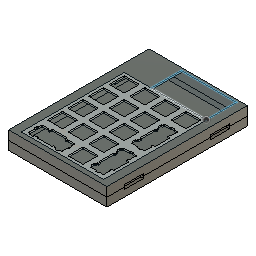
Keypad_case_top.glb (Autodesk Fusion 360 design; units mm, degrees)
part number: 2026-03-14-15-34-49-794
Autodesk Fusion 360 part; units mm, degrees
sketch "plate-2026-03-14T12_30_48.616Z" plane through (0, 0, 0) normal (0, 0, 1) x (1, 0, 0)
  line L0 (3.025, -26.3375) -> (16.025, -26.3375)
  line L1 (3.025, -40.3375) -> (16.025, -40.3375)
  line L2 (2.525, -26.8375) -> (2.525, -39.8375)
  line L3 (16.525, -26.8375) -> (16.525, -39.8375)
  arc A0 (3.025, -26.3375) -> (2.525, -26.8375) centre (3.025, -26.8375) ccw
  arc A1 (16.525, -26.8375) -> (16.025, -26.3375) centre (16.025, -26.8375) ccw
  arc A2 (2.525, -39.8375) -> (3.025, -40.3375) centre (3.025, -39.8375) ccw
  arc A3 (16.025, -40.3375) -> (16.525, -39.8375) centre (16.025, -39.8375) ccw
  line L4 (22.075, -26.3375) -> (35.075, -26.3375)
  line L5 (22.075, -40.3375) -> (35.075, -40.3375)
  line L6 (21.575, -26.8375) -> (21.575, -39.8375)
  line L7 (35.575, -26.8375) -> (35.575, -39.8375)
  arc A4 (22.075, -26.3375) -> (21.575, -26.8375) centre (22.075, -26.8375) ccw
  arc A5 (35.575, -26.8375) -> (35.075, -26.3375) centre (35.075, -26.8375) ccw
  arc A6 (21.575, -39.8375) -> (22.075, -40.3375) centre (22.075, -39.8375) ccw
  arc A7 (35.075, -40.3375) -> (35.575, -39.8375) centre (35.075, -39.8375) ccw
  line L8 (41.125, -26.3375) -> (54.125, -26.3375)
  line L9 (41.125, -40.3375) -> (54.125, -40.3375)
  line L10 (40.625, -26.8375) -> (40.625, -39.8375)
  line L11 (54.625, -26.8375) -> (54.625, -39.8375)
  arc A8 (41.125, -26.3375) -> (40.625, -26.8375) centre (41.125, -26.8375) ccw
  arc A9 (54.625, -26.8375) -> (54.125, -26.3375) centre (54.125, -26.8375) ccw
  arc A10 (40.625, -39.8375) -> (41.125, -40.3375) centre (41.125, -39.8375) ccw
  arc A11 (54.125, -40.3375) -> (54.625, -39.8375) centre (54.125, -39.8375) ccw
  line L12 (60.175, -26.3375) -> (73.175, -26.3375)
  line L13 (60.175, -40.3375) -> (73.175, -40.3375)
  line L14 (59.675, -26.8375) -> (59.675, -39.8375)
  line L15 (73.675, -26.8375) -> (73.675, -39.8375)
  arc A12 (60.175, -26.3375) -> (59.675, -26.8375) centre (60.175, -26.8375) ccw
  arc A13 (73.675, -26.8375) -> (73.175, -26.3375) centre (73.175, -26.8375) ccw
  arc A14 (59.675, -39.8375) -> (60.175, -40.3375) centre (60.175, -39.8375) ccw
  arc A15 (73.175, -40.3375) -> (73.675, -39.8375) centre (73.175, -39.8375) ccw
  line L16 (3.025, -45.3875) -> (16.025, -45.3875)
  line L17 (3.025, -59.3875) -> (16.025, -59.3875)
  line L18 (2.525, -45.8875) -> (2.525, -58.8875)
  line L19 (16.525, -45.8875) -> (16.525, -58.8875)
  arc A16 (3.025, -45.3875) -> (2.525, -45.8875) centre (3.025, -45.8875) ccw
  arc A17 (16.525, -45.8875) -> (16.025, -45.3875) centre (16.025, -45.8875) ccw
  arc A18 (2.525, -58.8875) -> (3.025, -59.3875) centre (3.025, -58.8875) ccw
  arc A19 (16.025, -59.3875) -> (16.525, -58.8875) centre (16.025, -58.8875) ccw
  line L20 (22.075, -45.3875) -> (35.075, -45.3875)
  line L21 (22.075, -59.3875) -> (35.075, -59.3875)
  line L22 (21.575, -45.8875) -> (21.575, -58.8875)
  line L23 (35.575, -45.8875) -> (35.575, -58.8875)
  arc A20 (22.075, -45.3875) -> (21.575, -45.8875) centre (22.075, -45.8875) ccw
  arc A21 (35.575, -45.8875) -> (35.075, -45.3875) centre (35.075, -45.8875) ccw
  arc A22 (21.575, -58.8875) -> (22.075, -59.3875) centre (22.075, -58.8875) ccw
  arc A23 (35.075, -59.3875) -> (35.575, -58.8875) centre (35.075, -58.8875) ccw
  line L24 (41.125, -45.3875) -> (54.125, -45.3875)
  line L25 (41.125, -59.3875) -> (54.125, -59.3875)
  line L26 (40.625, -45.8875) -> (40.625, -58.8875)
  line L27 (54.625, -45.8875) -> (54.625, -58.8875)
  arc A24 (41.125, -45.3875) -> (40.625, -45.8875) centre (41.125, -45.8875) ccw
  arc A25 (54.625, -45.8875) -> (54.125, -45.3875) centre (54.125, -45.8875) ccw
  arc A26 (40.625, -58.8875) -> (41.125, -59.3875) centre (41.125, -58.8875) ccw
  arc A27 (54.125, -59.3875) -> (54.625, -58.8875) centre (54.125, -58.8875) ccw
  line L28 (73.675, -55.4125) -> (73.675, -68.4125)
  line L29 (59.675, -55.4125) -> (59.675, -68.4125)
  line L30 (73.175, -54.9125) -> (60.175, -54.9125)
  line L31 (73.175, -68.9125) -> (60.175, -68.9125)
  arc A28 (73.675, -55.4125) -> (73.175, -54.9125) centre (73.175, -55.4125) ccw
  arc A29 (73.175, -68.9125) -> (73.675, -68.4125) centre (73.175, -68.4125) ccw
  arc A30 (60.175, -54.9125) -> (59.675, -55.4125) centre (60.175, -55.4125) ccw
  arc A31 (59.675, -68.4125) -> (60.175, -68.9125) centre (60.175, -68.4125) ccw
  line L32 (72.3646, -47.1471) -> (72.3646, -52.8019)
  line L33 (71.8646, -53.3019) -> (71.5518, -53.3019)
  line L34 (71.5518, -53.3019) -> (71.5518, -61.9125)
  line L35 (60.8584, -61.9125) -> (60.8584, -53.8019)
  line L36 (60.3584, -53.3019) -> (60.071, -53.3019)
  line L37 (60.071, -53.3019) -> (60.071, -51.9985)
  line L38 (59.571, -51.4985) -> (59.4026, -51.4985)
  line L39 (58.9026, -50.9985) -> (58.9026, -48.9505)
  line L40 (59.4026, -48.4505) -> (59.571, -48.4505)
  line L41 (60.071, -47.9505) -> (60.071, -47.1471)
  line L42 (60.571, -46.6471) -> (65.667, -46.6471)
  line L43 (66.167, -46.1471) -> (66.167, -45.7835)
  line L44 (66.167, -45.7835) -> (68.461, -45.7835)
  line L45 (68.961, -46.2835) -> (68.961, -46.6471)
  line L46 (68.961, -46.6471) -> (71.8646, -46.6471)
  arc A32 (71.8646, -53.3019) -> (72.3646, -52.8019) centre (71.8646, -52.8019) ccw
  arc A33 (60.8584, -53.8019) -> (60.3584, -53.3019) centre (60.3584, -53.8019) ccw
  arc A34 (60.071, -51.9985) -> (59.571, -51.4985) centre (59.571, -51.9985) ccw
  arc A35 (58.9026, -50.9985) -> (59.4026, -51.4985) centre (59.4026, -50.9985) ccw
  arc A36 (59.4026, -48.4505) -> (58.9026, -48.9505) centre (59.4026, -48.9505) ccw
  arc A37 (59.571, -48.4505) -> (60.071, -47.9505) centre (59.571, -47.9505) ccw
  arc A38 (60.571, -46.6471) -> (60.071, -47.1471) centre (60.571, -47.1471) ccw
  arc A39 (65.667, -46.6471) -> (66.167, -46.1471) centre (65.667, -46.1471) ccw
  arc A40 (68.961, -46.2835) -> (68.461, -45.7835) centre (68.461, -46.2835) ccw
  arc A41 (72.3646, -47.1471) -> (71.8646, -46.6471) centre (71.8646, -47.1471) ccw
  line L47 (72.3646, -76.6779) -> (72.3646, -71.0231)
  line L48 (71.8646, -70.5231) -> (71.5518, -70.5231)
  line L49 (71.5518, -70.5231) -> (71.5518, -61.9125)
  line L50 (60.8584, -61.9125) -> (60.8584, -70.0231)
  line L51 (60.3584, -70.5231) -> (60.071, -70.5231)
  line L52 (60.071, -70.5231) -> (60.071, -71.8265)
  line L53 (59.571, -72.3265) -> (59.4026, -72.3265)
  line L54 (58.9026, -72.8265) -> (58.9026, -74.8745)
  line L55 (59.4026, -75.3745) -> (59.571, -75.3745)
  line L56 (60.071, -75.8745) -> (60.071, -76.6779)
  line L57 (60.571, -77.1779) -> (65.667, -77.1779)
  line L58 (66.167, -77.6779) -> (66.167, -78.0415)
  line L59 (66.167, -78.0415) -> (68.461, -78.0415)
  line L60 (68.961, -77.5415) -> (68.961, -77.1779)
  line L61 (68.961, -77.1779) -> (71.8646, -77.1779)
  arc A42 (72.3646, -71.0231) -> (71.8646, -70.5231) centre (71.8646, -71.0231) ccw
  arc A43 (60.3584, -70.5231) -> (60.8584, -70.0231) centre (60.3584, -70.0231) ccw
  arc A44 (59.571, -72.3265) -> (60.071, -71.8265) centre (59.571, -71.8265) ccw
  arc A45 (59.4026, -72.3265) -> (58.9026, -72.8265) centre (59.4026, -72.8265) ccw
  arc A46 (58.9026, -74.8745) -> (59.4026, -75.3745) centre (59.4026, -74.8745) ccw
  arc A47 (60.071, -75.8745) -> (59.571, -75.3745) centre (59.571, -75.8745) ccw
  arc A48 (60.071, -76.6779) -> (60.571, -77.1779) centre (60.571, -76.6779) ccw
  arc A49 (66.167, -77.6779) -> (65.667, -77.1779) centre (65.667, -77.6779) ccw
  arc A50 (68.461, -78.0415) -> (68.961, -77.5415) centre (68.461, -77.5415) ccw
  arc A51 (71.8646, -77.1779) -> (72.3646, -76.6779) centre (71.8646, -76.6779) ccw
  line L62 (3.025, -64.4375) -> (16.025, -64.4375)
  line L63 (3.025, -78.4375) -> (16.025, -78.4375)
  line L64 (2.525, -64.9375) -> (2.525, -77.9375)
  line L65 (16.525, -64.9375) -> (16.525, -77.9375)
  arc A52 (3.025, -64.4375) -> (2.525, -64.9375) centre (3.025, -64.9375) ccw
  arc A53 (16.525, -64.9375) -> (16.025, -64.4375) centre (16.025, -64.9375) ccw
  arc A54 (2.525, -77.9375) -> (3.025, -78.4375) centre (3.025, -77.9375) ccw
  arc A55 (16.025, -78.4375) -> (16.525, -77.9375) centre (16.025, -77.9375) ccw
  line L66 (22.075, -64.4375) -> (35.075, -64.4375)
  line L67 (22.075, -78.4375) -> (35.075, -78.4375)
  line L68 (21.575, -64.9375) -> (21.575, -77.9375)
  line L69 (35.575, -64.9375) -> (35.575, -77.9375)
  arc A56 (22.075, -64.4375) -> (21.575, -64.9375) centre (22.075, -64.9375) ccw
  arc A57 (35.575, -64.9375) -> (35.075, -64.4375) centre (35.075, -64.9375) ccw
  arc A58 (21.575, -77.9375) -> (22.075, -78.4375) centre (22.075, -77.9375) ccw
  arc A59 (35.075, -78.4375) -> (35.575, -77.9375) centre (35.075, -77.9375) ccw
  line L70 (41.125, -64.4375) -> (54.125, -64.4375)
  line L71 (41.125, -78.4375) -> (54.125, -78.4375)
  line L72 (40.625, -64.9375) -> (40.625, -77.9375)
  line L73 (54.625, -64.9375) -> (54.625, -77.9375)
  arc A60 (41.125, -64.4375) -> (40.625, -64.9375) centre (41.125, -64.9375) ccw
  arc A61 (54.625, -64.9375) -> (54.125, -64.4375) centre (54.125, -64.9375) ccw
  arc A62 (40.625, -77.9375) -> (41.125, -78.4375) centre (41.125, -77.9375) ccw
  arc A63 (54.125, -78.4375) -> (54.625, -77.9375) centre (54.125, -77.9375) ccw
  line L74 (3.025, -83.4875) -> (16.025, -83.4875)
  line L75 (3.025, -97.4875) -> (16.025, -97.4875)
  line L76 (2.525, -83.9875) -> (2.525, -96.9875)
  line L77 (16.525, -83.9875) -> (16.525, -96.9875)
  arc A64 (3.025, -83.4875) -> (2.525, -83.9875) centre (3.025, -83.9875) ccw
  arc A65 (16.525, -83.9875) -> (16.025, -83.4875) centre (16.025, -83.9875) ccw
  arc A66 (2.525, -96.9875) -> (3.025, -97.4875) centre (3.025, -96.9875) ccw
  arc A67 (16.025, -97.4875) -> (16.525, -96.9875) centre (16.025, -96.9875) ccw
  line L78 (22.075, -83.4875) -> (35.075, -83.4875)
  line L79 (22.075, -97.4875) -> (35.075, -97.4875)
  line L80 (21.575, -83.9875) -> (21.575, -96.9875)
  line L81 (35.575, -83.9875) -> (35.575, -96.9875)
  arc A68 (22.075, -83.4875) -> (21.575, -83.9875) centre (22.075, -83.9875) ccw
  arc A69 (35.575, -83.9875) -> (35.075, -83.4875) centre (35.075, -83.9875) ccw
  arc A70 (21.575, -96.9875) -> (22.075, -97.4875) centre (22.075, -96.9875) ccw
  arc A71 (35.075, -97.4875) -> (35.575, -96.9875) centre (35.075, -96.9875) ccw
  line L82 (41.125, -83.4875) -> (54.125, -83.4875)
  line L83 (41.125, -97.4875) -> (54.125, -97.4875)
  line L84 (40.625, -83.9875) -> (40.625, -96.9875)
  line L85 (54.625, -83.9875) -> (54.625, -96.9875)
  arc A72 (41.125, -83.4875) -> (40.625, -83.9875) centre (41.125, -83.9875) ccw
  arc A73 (54.625, -83.9875) -> (54.125, -83.4875) centre (54.125, -83.9875) ccw
  arc A74 (40.625, -96.9875) -> (41.125, -97.4875) centre (41.125, -96.9875) ccw
  arc A75 (54.125, -97.4875) -> (54.625, -96.9875) centre (54.125, -96.9875) ccw
  line L86 (73.675, -93.5125) -> (73.675, -106.5125)
  line L87 (59.675, -93.5125) -> (59.675, -106.5125)
  line L88 (73.175, -93.0125) -> (60.175, -93.0125)
  line L89 (73.175, -107.0125) -> (60.175, -107.0125)
  arc A76 (73.675, -93.5125) -> (73.175, -93.0125) centre (73.175, -93.5125) ccw
  arc A77 (73.175, -107.0125) -> (73.675, -106.5125) centre (73.175, -106.5125) ccw
  arc A78 (60.175, -93.0125) -> (59.675, -93.5125) centre (60.175, -93.5125) ccw
  arc A79 (59.675, -106.5125) -> (60.175, -107.0125) centre (60.175, -106.5125) ccw
  line L90 (72.3646, -85.2471) -> (72.3646, -90.9019)
  line L91 (71.8646, -91.4019) -> (71.5518, -91.4019)
  line L92 (71.5518, -91.4019) -> (71.5518, -100.0125)
  line L93 (60.8584, -100.0125) -> (60.8584, -91.9019)
  line L94 (60.3584, -91.4019) -> (60.071, -91.4019)
  line L95 (60.071, -91.4019) -> (60.071, -90.0985)
  line L96 (59.571, -89.5985) -> (59.4026, -89.5985)
  line L97 (58.9026, -89.0985) -> (58.9026, -87.0505)
  line L98 (59.4026, -86.5505) -> (59.571, -86.5505)
  line L99 (60.071, -86.0505) -> (60.071, -85.2471)
  line L100 (60.571, -84.7471) -> (65.667, -84.7471)
  line L101 (66.167, -84.2471) -> (66.167, -83.8835)
  line L102 (66.167, -83.8835) -> (68.461, -83.8835)
  line L103 (68.961, -84.3835) -> (68.961, -84.7471)
  line L104 (68.961, -84.7471) -> (71.8646, -84.7471)
  arc A80 (71.8646, -91.4019) -> (72.3646, -90.9019) centre (71.8646, -90.9019) ccw
  arc A81 (60.8584, -91.9019) -> (60.3584, -91.4019) centre (60.3584, -91.9019) ccw
  arc A82 (60.071, -90.0985) -> (59.571, -89.5985) centre (59.571, -90.0985) ccw
  arc A83 (58.9026, -89.0985) -> (59.4026, -89.5985) centre (59.4026, -89.0985) ccw
  arc A84 (59.4026, -86.5505) -> (58.9026, -87.0505) centre (59.4026, -87.0505) ccw
  arc A85 (59.571, -86.5505) -> (60.071, -86.0505) centre (59.571, -86.0505) ccw
  arc A86 (60.571, -84.7471) -> (60.071, -85.2471) centre (60.571, -85.2471) ccw
  arc A87 (65.667, -84.7471) -> (66.167, -84.2471) centre (65.667, -84.2471) ccw
  arc A88 (68.961, -84.3835) -> (68.461, -83.8835) centre (68.461, -84.3835) ccw
  arc A89 (72.3646, -85.2471) -> (71.8646, -84.7471) centre (71.8646, -85.2471) ccw
  line L105 (72.3646, -114.7779) -> (72.3646, -109.1231)
  line L106 (71.8646, -108.6231) -> (71.5518, -108.6231)
  line L107 (71.5518, -108.6231) -> (71.5518, -100.0125)
  line L108 (60.8584, -100.0125) -> (60.8584, -108.1231)
  line L109 (60.3584, -108.6231) -> (60.071, -108.6231)
  line L110 (60.071, -108.6231) -> (60.071, -109.9265)
  line L111 (59.571, -110.4265) -> (59.4026, -110.4265)
  line L112 (58.9026, -110.9265) -> (58.9026, -112.9745)
  line L113 (59.4026, -113.4745) -> (59.571, -113.4745)
  line L114 (60.071, -113.9745) -> (60.071, -114.7779)
  line L115 (60.571, -115.2779) -> (65.667, -115.2779)
  line L116 (66.167, -115.7779) -> (66.167, -116.1415)
  line L117 (66.167, -116.1415) -> (68.461, -116.1415)
  line L118 (68.961, -115.6415) -> (68.961, -115.2779)
  line L119 (68.961, -115.2779) -> (71.8646, -115.2779)
  arc A90 (72.3646, -109.1231) -> (71.8646, -108.6231) centre (71.8646, -109.1231) ccw
  arc A91 (60.3584, -108.6231) -> (60.8584, -108.1231) centre (60.3584, -108.1231) ccw
  arc A92 (59.571, -110.4265) -> (60.071, -109.9265) centre (59.571, -109.9265) ccw
  arc A93 (59.4026, -110.4265) -> (58.9026, -110.9265) centre (59.4026, -110.9265) ccw
  arc A94 (58.9026, -112.9745) -> (59.4026, -113.4745) centre (59.4026, -112.9745) ccw
  arc A95 (60.071, -113.9745) -> (59.571, -113.4745) centre (59.571, -113.9745) ccw
  arc A96 (60.071, -114.7779) -> (60.571, -115.2779) centre (60.571, -114.7779) ccw
  arc A97 (66.167, -115.7779) -> (65.667, -115.2779) centre (65.667, -115.7779) ccw
  arc A98 (68.461, -116.1415) -> (68.961, -115.6415) centre (68.461, -115.6415) ccw
  arc A99 (71.8646, -115.2779) -> (72.3646, -114.7779) centre (71.8646, -114.7779) ccw
  line L120 (12.55, -102.5375) -> (25.55, -102.5375)
  line L121 (12.55, -116.5375) -> (25.55, -116.5375)
  line L122 (12.05, -103.0375) -> (12.05, -116.0375)
  line L123 (26.05, -103.0375) -> (26.05, -116.0375)
  arc A100 (12.55, -102.5375) -> (12.05, -103.0375) centre (12.55, -103.0375) ccw
  arc A101 (26.05, -103.0375) -> (25.55, -102.5375) centre (25.55, -103.0375) ccw
  arc A102 (12.05, -116.0375) -> (12.55, -116.5375) centre (12.55, -116.0375) ccw
  arc A103 (25.55, -116.5375) -> (26.05, -116.0375) centre (25.55, -116.0375) ccw
  line L124 (4.2846, -103.8479) -> (9.9394, -103.8479)
  line L125 (10.4394, -104.3479) -> (10.4394, -104.6607)
  line L126 (10.4394, -104.6607) -> (19.05, -104.6607)
  line L127 (19.05, -115.3541) -> (10.9394, -115.3541)
  line L128 (10.4394, -115.8541) -> (10.4394, -116.1415)
  line L129 (10.4394, -116.1415) -> (9.136, -116.1415)
  line L130 (8.636, -116.6415) -> (8.636, -116.8099)
  line L131 (8.136, -117.3099) -> (6.088, -117.3099)
  line L132 (5.588, -116.8099) -> (5.588, -116.6415)
  line L133 (5.088, -116.1415) -> (4.2846, -116.1415)
  line L134 (3.7846, -115.6415) -> (3.7846, -110.5455)
  line L135 (3.2846, -110.0455) -> (2.921, -110.0455)
  line L136 (2.921, -110.0455) -> (2.921, -107.7515)
  line L137 (3.421, -107.2515) -> (3.7846, -107.2515)
  line L138 (3.7846, -107.2515) -> (3.7846, -104.3479)
  arc A104 (10.4394, -104.3479) -> (9.9394, -103.8479) centre (9.9394, -104.3479) ccw
  arc A105 (10.9394, -115.3541) -> (10.4394, -115.8541) centre (10.9394, -115.8541) ccw
  arc A106 (9.136, -116.1415) -> (8.636, -116.6415) centre (9.136, -116.6415) ccw
  arc A107 (8.136, -117.3099) -> (8.636, -116.8099) centre (8.136, -116.8099) ccw
  arc A108 (5.588, -116.8099) -> (6.088, -117.3099) centre (6.088, -116.8099) ccw
  arc A109 (5.588, -116.6415) -> (5.088, -116.1415) centre (5.088, -116.6415) ccw
  arc A110 (3.7846, -115.6415) -> (4.2846, -116.1415) centre (4.2846, -115.6415) ccw
  arc A111 (3.7846, -110.5455) -> (3.2846, -110.0455) centre (3.2846, -110.5455) ccw
  arc A112 (3.421, -107.2515) -> (2.921, -107.7515) centre (3.421, -107.7515) ccw
  arc A113 (4.2846, -103.8479) -> (3.7846, -104.3479) centre (4.2846, -104.3479) ccw
  line L139 (33.8154, -103.8479) -> (28.1606, -103.8479)
  line L140 (27.6606, -104.3479) -> (27.6606, -104.6607)
  line L141 (27.6606, -104.6607) -> (19.05, -104.6607)
  line L142 (19.05, -115.3541) -> (27.1606, -115.3541)
  line L143 (27.6606, -115.8541) -> (27.6606, -116.1415)
  line L144 (27.6606, -116.1415) -> (28.964, -116.1415)
  line L145 (29.464, -116.6415) -> (29.464, -116.8099)
  line L146 (29.964, -117.3099) -> (32.012, -117.3099)
  line L147 (32.512, -116.8099) -> (32.512, -116.6415)
  line L148 (33.012, -116.1415) -> (33.8154, -116.1415)
  line L149 (34.3154, -115.6415) -> (34.3154, -110.5455)
  line L150 (34.8154, -110.0455) -> (35.179, -110.0455)
  line L151 (35.179, -110.0455) -> (35.179, -107.7515)
  line L152 (34.679, -107.2515) -> (34.3154, -107.2515)
  line L153 (34.3154, -107.2515) -> (34.3154, -104.3479)
  arc A114 (28.1606, -103.8479) -> (27.6606, -104.3479) centre (28.1606, -104.3479) ccw
  arc A115 (27.6606, -115.8541) -> (27.1606, -115.3541) centre (27.1606, -115.8541) ccw
  arc A116 (29.464, -116.6415) -> (28.964, -116.1415) centre (28.964, -116.6415) ccw
  arc A117 (29.464, -116.8099) -> (29.964, -117.3099) centre (29.964, -116.8099) ccw
  arc A118 (32.012, -117.3099) -> (32.512, -116.8099) centre (32.012, -116.8099) ccw
  arc A119 (33.012, -116.1415) -> (32.512, -116.6415) centre (33.012, -116.6415) ccw
  arc A120 (33.8154, -116.1415) -> (34.3154, -115.6415) centre (33.8154, -115.6415) ccw
  arc A121 (34.8154, -110.0455) -> (34.3154, -110.5455) centre (34.8154, -110.5455) ccw
  arc A122 (35.179, -107.7515) -> (34.679, -107.2515) centre (34.679, -107.7515) ccw
  arc A123 (34.3154, -104.3479) -> (33.8154, -103.8479) centre (33.8154, -104.3479) ccw
  line L154 (41.125, -102.5375) -> (54.125, -102.5375)
  line L155 (41.125, -116.5375) -> (54.125, -116.5375)
  line L156 (40.625, -103.0375) -> (40.625, -116.0375)
  line L157 (54.625, -103.0375) -> (54.625, -116.0375)
  arc A124 (41.125, -102.5375) -> (40.625, -103.0375) centre (41.125, -103.0375) ccw
  arc A125 (54.625, -103.0375) -> (54.125, -102.5375) centre (54.125, -103.0375) ccw
  arc A126 (40.625, -116.0375) -> (41.125, -116.5375) centre (41.125, -116.0375) ccw
  arc A127 (54.125, -116.5375) -> (54.625, -116.0375) centre (54.125, -116.0375) ccw
  line L158 (0, -119.0625) -> (76.2, -119.0625)
  line L159 (0, -23.8125) -> (76.2, -23.8125)
  line L160 (0, -119.0625) -> (0, -23.8125)
  line L161 (76.2, -119.0625) -> (76.2, -23.8125)
extrude "Extrude1" add sketch "plate-2026-03-14T12_30_48.616Z" along normal blind 1.5 makes body 1
extrude "Extrude16" add 1 faces at (76.2, -87.3125, 0.5) along direction (1, 0, 0) blind 5 separate body on bodies 1 makes body 2
extrude "Extrude17" add 1 faces at (0, -87.3125, 0.5) along direction (-1, 0, 0) blind 5 separate body on bodies 1 makes body 3
extrude "Extrude18" add 3 faces at (25.4, -119.0625, 1) (77.8667, -119.0625, 0.5) (-1.6667, -119.0625, 0.5) along direction (0, -1, 0) blind 1 separate body on bodies 1 2 3 makes body 4
extrude "Extrude19" add 1 faces at (25.4, -120.0625, 1) along direction (0, -1, 0) blind 1 on bodies 4 bodies 4
combine "Combine1" operation add target body 2 tool bodies 3 4
extrude "Extrude20" add 3 faces at (25.4, -23.8125, 1) (-1.6667, -23.8125, 0.5) (77.8667, -23.8125, 0.5) along direction (0, 1, 0) blind 28 separate body on bodies 1 2 makes body 5
combine "Combine2" operation add target body 5 tool bodies 2
sketch "Sketch4" plane through (0, 0, 0) normal (0, 0, 1) x (1, 0, 0)
  line L0 (0, 0) -> (86, 0)
  line L1 (86, 0) -> (86, -125)
  line L2 (86, -125) -> (0, -125)
  line L3 (0, -125) -> (0, 0)
  line L4 (-2.5, 2.5) -> (88.5, 2.5)
  line L5 (88.5, 2.5) -> (88.5, -127.5)
  line L6 (88.5, -127.5) -> (-2.5, -127.5)
  line L7 (-2.5, -127.5) -> (-2.5, 2.5)
  dimension "d44" = 86
  dimension "d45" = 125
  dimension "d46" = 2.5
  dimension "d47" = 2.5
  dimension "d48" = 2.5
  dimension "d49" = 2.5
  constraint horizontal L0
  constraint vertical L1
  constraint horizontal L2
  constraint vertical L3
  constraint coincident L0.start L3.end
  constraint horizontal L4
  constraint vertical L5
  constraint horizontal L6
  constraint vertical L7
  measures "d44" distance of L0.start L0.end
  measures "d45" distance of L0.start L2.end
  measures "d46" distance of L3 L7
  measures "d47" distance of L0 L4
  measures "d48" distance of L1 L5
  measures "d49" distance of L2 L6
move_body "Move1" bodies 5 1 to x (1, 0, 0) y (0, 1, 0) z (0, 0, 1) at (5, -4.1875, 0)
extrude "Extrude21" add sketch "Sketch4" against normal blind 7 separate body makes body 6
extrude "Extrude22" add 1 faces at (-1.6667, -83.3333, 0) along direction (0, 0, 1) blind 1.5 on bodies 6 bodies 5 6
extrude "Extrude23" add sketch "Sketch4" along normal blind 3 separate body contours L0 L1 L2 L3 | L4 L5 L6 L7 makes body 7
extrude "Extrude24" add sketch "Sketch4" along normal blind 10 bodies 7
extrude "Extrude25" cut 1 faces at (-1.6667, -83.3333, 10) along direction (0, 0, -1) blind 5 on bodies 7 bodies 7
extrude "Extrude26" add 1 faces at (-1.6667, -83.3333, 5) along direction (0, 0, 1) blind 3 on bodies 7 bodies 7
move_body "Move2" bodies 7 to x (1, 0, 0) y (0, 1, 0) z (0, 0, 1) at (0, 0, -13)
move_body "Move3" bodies 7 to x (1, 0, 0) y (0, 1, 0) z (0, 0, 1) at (0, 0, -2)
sketch "Sketch5" plane through (0, 0, 1.5) normal (0, 0, 1) x (-1, 0, 0)
  line L0 (2.5, 127.5) -> (-88.5, 127.5)
  line L1 (-88.5, 127.5) -> (-88.5, -2.5)
  line L2 (-88.5, -2.5) -> (2.5, -2.5)
  line L3 (2.5, -2.5) -> (2.5, 127.5)
  line L4 (-5, 28) -> (-81.2, 28)
  line L5 (-81.2, 28) -> (-81.2, 123.25)
  line L6 (-81.2, 123.25) -> (-5, 123.25)
  line L7 (-5, 123.25) -> (-5, 28)
  line L8 (-30, 0) -> (-81, 0)
  line L9 (-81, 0) -> (-81, 28)
  line L10 (-81, 28) -> (-30, 28)
  line L11 (-30, 28) -> (-30, 0)
  constraint horizontal L8
  constraint vertical L9
  constraint horizontal L10
  constraint vertical L11
  constraint coincident L4 L9.end
extrude "Extrude27" cut sketch "Sketch5" against normal blind 2 contours L4 L8 L9 L10 L11 bodies 5
sketch "Sketch6" plane through (88.5, 0, 0) normal (1, 0, 0) x (0, 1, 0)
  line L0 (-127.5, -7) -> (-127.5, -15)
  line L1 (-127.5, -15) -> (2.5, -15)
  line L2 (2.5, -15) -> (2.5, -7)
  line L3 (2.5, -7) -> (-127.5, -7)
  line L4 (-111, -4.91) -> (-93.5, -4.91)
  line L5 (-93.5, -4.91) -> (-93.5, -8.91)
  line L6 (-93.5, -8.91) -> (-111, -8.91)
  line L7 (-111, -8.91) -> (-111, -4.91)
  line L8 (-31.5, -4.91) -> (-14, -4.91)
  line L9 (-14, -4.91) -> (-14, -8.91)
  line L10 (-14, -8.91) -> (-31.5, -8.91)
  line L11 (-31.5, -8.91) -> (-31.5, -4.91)
  dimension "d64" = 4
  dimension "d65" = 17.5
  dimension "d66" = 16.5
  dimension "d67" = 6.09
  dimension "d68" = 4
  dimension "d69" = 17.5
  dimension "d71" = 16.5
  constraint horizontal L4
  constraint vertical L5
  constraint horizontal L6
  constraint vertical L7
  constraint horizontal L8
  constraint vertical L9
  constraint horizontal L10
  constraint vertical L11
  measures "d64" distance of L4.start L6.end
  measures "d65" distance of L4.start L4.end
  measures "d66" distance of L0 L7
  measures "d67" distance of L1 L6
  measures "d68" distance of L10.end L8.start
  measures "d69" distance of L8.end L8.start
  measures "d71" distance of L2 L9
extrude "Extrude28" cut sketch "Sketch6" against normal blind 91 contours L3 L4 L5 L7 | L3 L5 L6 L7 | L3 L8 L9 L11 | L3 L9 L10 L11 bodies 5 7
sketch "Sketch8" plane through (0, 2.5, 0) normal (0, 1, 0) x (-1, 0, 0)
  line L0 (-88.5, 1.5) -> (-88.5, -7)
  line L1 (-88.5, -7) -> (2.5, -7)
  line L2 (2.5, -7) -> (2.5, 1.5)
  line L3 (2.5, 1.5) -> (-88.5, 1.5)
  line L4 (-19.25, -5.5) -> (-9.25, -5.5)
  line L5 (-9.25, -5.5) -> (-9.25, -10)
  line L6 (-9.25, -10) -> (-19.25, -10)
  line L7 (-19.25, -10) -> (-19.25, -5.5)
  line L8 (2.5, -15) -> (-88.5, -15)
  dimension "d81" = 5
  dimension "d82" = 11.75
  dimension "d83" = 4.5
  dimension "d84" = 10
  constraint horizontal L4
  constraint vertical L5
  constraint horizontal L6
  constraint vertical L7
  measures "d81" distance of L6 L8
  measures "d82" distance of L2 L5
  measures "d83" distance of L4 L6
  measures "d84" distance of L5 L7
extrude "Extrude30" cut sketch "Sketch8" against normal blind 4 contours L1 L4 L5 L7 | L1 L5 L6 L7 bodies 5 7
extrude "Extrude29" [suppressed]
